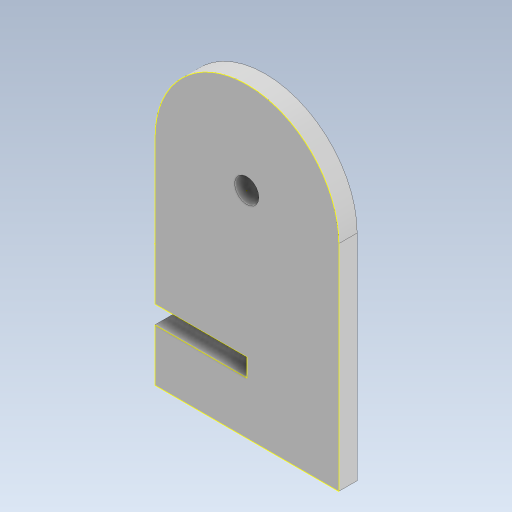
# Autodesk Inventor part: 零件7
Saved by Autodesk Inventor 2023 (Build 270158000, 158)
## iProperties
Created: 2023-05-12
Part Number: 零件7
Material: 一般
Document SubType Name: Modeling
Designer: Johnny Jou
Density: 1 g/cm^3
Appearance: 預設
Author: Johnny Jou
Autodesk Inventor part; units mm, degrees
ref_plane "YZ Plane" through (0, 0, 0) normal (1, 0, 0) x (0, 1, 0)
ref_plane "XZ Plane" through (0, 0, 0) normal (0, 1, 0) x (-1, 0, 0)
ref_plane "XY Plane" through (0, 0, 0) normal (0, 0, 1) x (1, 0, 0)
sketch "草圖1" plane through (0, 0, 0) normal (0, 0, 1) x (1, 0, 0)
  line L0 (0, 0) -> (15, 0)
  line L1 (15, -20) -> (0, -20)
  line L2 (0, -20) -> (0, 0)
  line L3 (0, -8.525) -> (15, -8.525)
  line L4 (15, -8.525) -> (15, -11.475)
  line L5 (15, -11.475) -> (0, -11.475)
  line L6 (0, -11.475) -> (0, -8.525)
  line L7 (15, 0) -> (60, 0)
  line L8 (15, 0) -> (15, -20)
  line L9 (15, -20) -> (30, -20)
  circle A0 centre (15, 15) radius 1.975
  circle A1 centre (15, 15) radius 15
  line L10 (30, -20) -> (30, 0)
  line L11 (15, 0) -> (15, -20)
  line L12 (0, 0) -> (0, 15)
  line L13 (30, 0) -> (30, 15)
  point P0 (15, -10)
  point P1 (0, -10)
  point P2 (15, 0)
  dimension "d0" = 20
  dimension "d3" = 2.95
  dimension "d4" = 0
  dimension "d7" = 15
  dimension "d9" = 3.95
  dimension "d15" = 15
  dimension "d16" = 30
  constraints: 28 end point, 4 horizontal, 4 parallel, 4 tangent, 3 perpendicular, 3 point on line, 2 centre point, 2 midpoint, 2 point on circle, 1 coincident, 1 collinear
  measures "d0" distance between parallel lines of L1 L0
  measures "d3" distance of L3.end L4.end
  measures "d4" vertical distance of point (15, -10) point (0, -10)
  measures "d7" distance between parallel lines of L2 L8
  measures "d9" diameter of A0
  measures "d15" distance between parallel lines of L10 L8
  measures "d16" diameter of A1
extrude "擠出1" add sketch "草圖1" along normal blind 3 contours L12 A1 L0 | L0 L8 L3 L2 | A1 L13 L7 | L7 L10 L9 L8 L4 | A1 | L5 L8 L1 L2
sketch "草圖2" plane through (0, 0, 3) normal (0, 0, 1) x (1, 0, 0)
  line L0 (0, -20) -> (30, -20) projected
  line L1 (0, 15) -> (0, -8.525) projected
  arc A0 (30, 15) -> (0, 15) centre (15, 15) ccw projected
  line L2 (30, -20) -> (30, 15) projected
  line L3 (0, -8.525) -> (15, -8.525) projected
  line L4 (15, -8.525) -> (15, -11.475) projected
  line L5 (15, -11.475) -> (0, -11.475) projected
  line L6 (0, -11.475) -> (0, -20) projected
  point P0 (0, 0)
